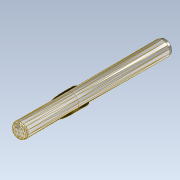
# Autodesk Inventor part: boquilla_flauta1
Saved by Autodesk Inventor 2022 (Build 260153000, 153)
## iProperties
Created: 2022-11-16
Part Number: boquilla_flauta1
Material: Generic
Document SubType Name: Modeling
Designer: ferna
Density: 1 g/cm^3
Appearance: Galvanized
Author: ferna
Autodesk Inventor part; units mm, degrees
ref_plane "YZ Plane" through (0, 0, 0) normal (1, 0, 0) x (0, 1, 0)
ref_plane "XY Plane" through (0, 0, 0) normal (0, 0, 1) x (1, 0, 0)
imported_surface "MeshFeature1"
ref_plane "Work Plane1" through (-2.6106, 2.6297, 220.7524) normal (0, 1, 0) x (-1, 0, 0)
sketch "Sketch1" plane through (1.1831, -10.543, 132.316) normal (0, 0, -1) x (-0.9946942, -0.1028758, 0)
  line L0 (-2.5151, 11.1045) -> (-0.3324, 12.9405) projected
  line L1 (7.1683, 0.7423) -> (9.2884, 2.5827) projected
  line L2 (-2.3794, 1.8172) -> (-2.9389, 3.1648) projected
  line L3 (5.8752, 13.2951) -> (8.2554, 11.756) projected
  circle A0 centre (3.1551, 6.6281) radius 7.0756
  circle A1 centre (3.1551, 6.6281) radius 6.4364
  point P0 (0.0922, 10.6088)
  constraints: 3 tangent, 2 centre point, 1 coincident
extrude "Extrusion1" add sketch "Sketch1" along normal blind 2.54 contours A1
sketch "Sketch2" plane through (-2.6371, -4.2747, 129.776) normal (0, 0, -1) x (-1, 0, 0)
  circle A0 centre (0, 0) radius 6.4364 projected
  circle A1 centre (0, 0) radius 5.9144
  line L0 (5.8742, 1.254) -> (4.4896, 4.6636) projected
  point P0 (-2.6371, 4.2747)
  constraints: 1 centre point, 1 coincident, 1 tangent
extrude "Extrusion2" cut sketch "Sketch2" against normal blind 137.4775 contours A1
body "Solid1"
body "Srf1"
